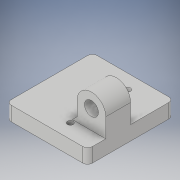
# Autodesk Inventor part: Mount for TMP007 Sensor
Saved by Autodesk Inventor 2018 (Build 220112000, 112)
## iProperties
Created: 2018-10-23
Part Number: Mount for TMP007 Sensor
Material: Generic
Document SubType Name: Modeling
Designer: tbrow
Density: 1 g/cm^3
Appearance: Default
Author: tbrow
## iProperties of the stored document Mount for TMP007 Sensor_3DPrint.ipt
Created: 2019-01-15
Part Number: Mount for TMP007 Sensor_3DPrint
Material: Generic
Document SubType Name: Modeling
Designer: tbrow
Density: 1 g/cm^3
Appearance: Default
Author: tbrow
Autodesk Inventor part; units mm, degrees
ref_plane "YZ Plane" through (0, 0, 0) normal (1, 0, 0) x (0, 1, 0)
ref_plane "XZ Plane" through (0, 0, 0) normal (0, 1, 0) x (-1, 0, 0)
ref_plane "XY Plane" through (0, 0, 0) normal (0, 0, 1) x (1, 0, 0)
sketch "Sketch1" plane through (0, 0, 0) normal (0, 1, 0) x (-1, 0, 0)
  line L0 (0, 0) -> (21.59, 0)
  line L1 (21.59, 0) -> (21.59, -22.86)
  line L2 (21.59, -22.86) -> (0, -22.86)
  line L3 (0, -22.86) -> (0, 0)
  line L4 (6.35, 0) -> (6.35, -22.86) construction
  circle A0 centre (8.382, -3.7846) radius 0.762
  circle A1 centre (8.382, -19.0754) radius 0.762
  line L5 (6.35, -3.7846) -> (7.62, -3.7846) construction
  line L6 (8.382, -3.0226) -> (8.382, 0) construction
  line L7 (7.62, -19.0754) -> (6.35, -19.0754) construction
  line L8 (8.382, -19.8374) -> (8.382, -22.86) construction
  line L9 (17.653, -10.287) -> (15.367, -10.287) construction
  line L10 (15.367, -10.287) -> (15.367, -12.573) construction
  line L11 (15.367, -12.573) -> (17.653, -12.573) construction
  line L12 (17.653, -12.573) -> (17.653, -10.287) construction
  line L13 (17.653, -11.43) -> (15.367, -11.43) construction
  line L14 (16.51, -10.287) -> (16.51, -12.573) construction
  line L15 (8.382, -19.0754) -> (8.382, -3.7846) construction
  point P0 (6.35, -11.43)
  dimension "d0" = 22.86
  dimension "d1" = 21.59
  dimension "d2" = 1.524
  dimension "d3" = 1.524
  dimension "d4" = 1.27
  dimension "d6" = 1.27
  dimension "d10" = 15.24
  dimension "d11" = 2.286
  dimension "d12" = 2.286
  dimension "d13" = 10.16
  dimension "d14" = 16.51
  dimension "d30" = 15.2908
  dimension "d31" = 3.0226
  constraints: 32 end point, 11 point on line, 7 perpendicular, 5 midpoint, 4 parallel, 4 point on circle, 2 centre point, 2 horizontal
  measures "d0" distance of L2.end L0.start
  measures "d1" distance of L1.end L2.end
  measures "d2" diameter of A0
  measures "d3" diameter of A1
  measures "d4" distance of L5.start L5.end
  measures "d6" distance of L7.start L7.end
  measures "d10" distance between parallel lines of L1 L4
  measures "d11" distance of L11.end L9.start
  measures "d12" distance of L10.end L11.end
  measures "d13" distance between parallel lines of L4 L14
  measures "d14" distance between parallel lines of L3 L14
  measures "d30" distance of L15.start L15.end
  measures "d31" distance of L8.start L8.end
extrude "Extrusion1" add sketch "Sketch1" along normal blind 3.81
sketch "Sketch2" plane through (0, 3.81, 0) normal (0, 1, 0) x (1, 0, 0)
  line L0 (-21.59, 22.86) -> (-21.59, 0) projected
  line L1 (-21.59, 11.43) -> (0, 11.43) construction
  line L2 (0, 0) -> (0, 22.86) projected
  line L3 (0, 11.43) -> (-7.62, 11.43)
  line L4 (-7.62, 11.43) -> (-7.62, 4.826)
  line L5 (-7.62, 4.826) -> (0, 4.826)
  line L6 (0, 4.826) -> (0, 11.43)
  dimension "d17" = 6.604
  dimension "d18" = 7.62
  constraints: 10 end point, 2 midpoint, 2 parallel, 1 horizontal, 1 perpendicular
  measures "d17" distance of L3.end L4.end
  measures "d18" distance of L4.end L5.end
extrude "Extrusion2" add sketch "Sketch2" along normal blind 8.89
fillet "Fillet1" radius 3.81 2 edges at (-7.62, 12.7, -8.128) (0, 12.7, -8.128)
sketch "Sketch3" plane through (-7.62, 3.81, -4.826) normal (0, 0, 1) x (1, 0, 0)
  arc A0 (7.62, 5.08) -> (0, 5.08) centre (3.81, 5.08) ccw projected
  circle A1 centre (3.81, 5.08) radius 1.8542
  point P0 (7.62, -3.81)
  dimension "d22" = 3.7084
  constraints: 1 centre point, 1 coincident
  measures "d22" diameter of A1
extrude "Extrusion4" cut sketch "Sketch3" against normal through all
chamfer "Chamfer1" distance 1.27 angle 45 1 edges at (-7.62, 3.81, -8.128)
fillet "Fillet2" radius 1.27 4 edges at (-21.59, 1.905, 0) (0, 1.905, 0) (0, 1.905, -22.86) (-21.59, 1.905, -22.86)
equation "\"d3\" = d2"
equation "\"d6\" = d4"
equation "\"d31\" = -0.5 * d2 + 0.5 * d0 - 0.5 * d30"
body "Solid1"
